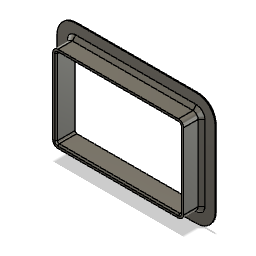
Power_Meter_Shield v1 (Autodesk Fusion 360 design; units mm, degrees)
Autodesk Fusion 360 part; units mm, degrees
sketch "Sketch1" plane through (0, 0, 0) normal (0, 0, 1) x (1, 0, 0)
  line L0 (36, -22.85) -> (-36, -22.85) construction
  line L1 (-36, -22.85) -> (-36, 22.85) construction
  line L2 (-36, 22.85) -> (36, 22.85) construction
  line L3 (36, 22.85) -> (36, -22.85) construction
  line L4 (36, -22.85) -> (-36, 22.85) construction
  line L5 (-36, -22.85) -> (36, 22.85) construction
  line L6 (35.3, -23.15) -> (-35.3, -23.15)
  line L7 (-36.3, -22.15) -> (-36.3, 22.15)
  line L8 (-35.3, 23.15) -> (35.3, 23.15)
  line L9 (36.3, 22.15) -> (36.3, -22.15)
  arc A0 (-35.3, 23.15) -> (-36.3, 22.15) centre (-35.3, 22.15) ccw
  arc A1 (35.3, -23.15) -> (36.3, -22.15) centre (35.3, -22.15) ccw
  arc A2 (36.3, 22.15) -> (35.3, 23.15) centre (35.3, 22.15) ccw
  arc A3 (-36.3, -22.15) -> (-35.3, -23.15) centre (-35.3, -22.15) ccw
  arc A4 (38.3, 22.15) -> (35.3, 25.15) centre (35.3, 22.15) ccw
  line L10 (-35.3, 25.15) -> (35.3, 25.15)
  arc A5 (-35.3, 25.15) -> (-38.3, 22.15) centre (-35.3, 22.15) ccw
  line L11 (-38.3, -22.15) -> (-38.3, 22.15)
  arc A6 (-38.3, -22.15) -> (-35.3, -25.15) centre (-35.3, -22.15) ccw
  line L12 (35.3, -25.15) -> (-35.3, -25.15)
  arc A7 (35.3, -25.15) -> (38.3, -22.15) centre (35.3, -22.15) ccw
  line L13 (38.3, 22.15) -> (38.3, -22.15)
  arc A8 (46.3, 22.15) -> (35.3, 33.15) centre (35.3, 22.15) ccw
  line L14 (-35.3, 33.15) -> (35.3, 33.15)
  arc A9 (-35.3, 33.15) -> (-46.3, 22.15) centre (-35.3, 22.15) ccw
  line L15 (-46.3, -22.15) -> (-46.3, 22.15)
  arc A10 (-46.3, -22.15) -> (-35.3, -33.15) centre (-35.3, -22.15) ccw
  line L16 (35.3, -33.15) -> (-35.3, -33.15)
  arc A11 (35.3, -33.15) -> (46.3, -22.15) centre (35.3, -22.15) ccw
  line L17 (46.3, 22.15) -> (46.3, -22.15)
  dimension "d3" = 45.7
  dimension "d4" = 72
  dimension "d6" = 1
  dimension "d7" = -2
  dimension "d8" = -10
  constraint horizontal L0
  constraint perpendicular L0 L1
  constraint parallel L0 L2
  constraint parallel L1 L3
  constraint coincident L4 origin
  constraint coincident L5 origin
  constraint tangent L7 A0
  constraint tangent L8 A0
  constraint tangent L6 A1
  constraint tangent L9 A1
  constraint equal A0 A1
  constraint tangent L8 A2
  constraint tangent L9 A2
  constraint equal A0 A2
  constraint tangent L6 A3
  constraint tangent L7 A3
  constraint equal A0 A3
  measures "d3" distance of L0.start L2.end
  measures "d4" distance of L0.start L0.end
  measures "d6" radius of A0
  measures "d7" distance of A2
extrude "Extrude1" add sketch "Sketch1" along normal blind 11.5 contours A4 L10 A5 L11 A6 L12 A7 L13
extrude "Extrude2" add sketch "Sketch1" along normal blind 1 contours A8 L14 A9 L15 A10 L16 A11 L17
chamfer "Chamfer1" distance 0.8 angle 45 8 edges at (0, 23.15, 11.5) (36.0071, 22.8571, 11.5) (36.3, 0, 11.5) (36.0071, -22.8571, 11.5) (0, -23.15, 11.5) (-36.0071, -22.8571, 11.5) (-36.3, 0, 11.5) (-36.0071, 22.8571, 11.5)
chamfer "Chamfer2" distance 2 angle 45 8 edges at (0, 25.15, 1) (-37.4213, 24.2713, 1) (-38.3, 0, 1) (-37.4213, -24.2713, 1) (0, -25.15, 1) (37.4213, -24.2713, 1) (38.3, 0, 1) (37.4213, 24.2713, 1)
chamfer "Chamfer3" distance 0.5 angle 45 16 edges at (0, 33.15, 0) (43.0782, 29.9282, 0) (46.3, 0, 0) (43.0782, -29.9282, 0) (0, -33.15, 0) (-43.0782, -29.9282, 0) (-46.3, 0, 0) (-43.0782, 29.9282, 0) (0, 23.15, 0) (36.0071, 22.8571, 0) (36.3, 0, 0) (36.0071, -22.8571, 0) (0, -23.15, 0) (-36.0071, -22.8571, 0) (-36.3, 0, 0) (-36.0071, 22.8571, 0)
